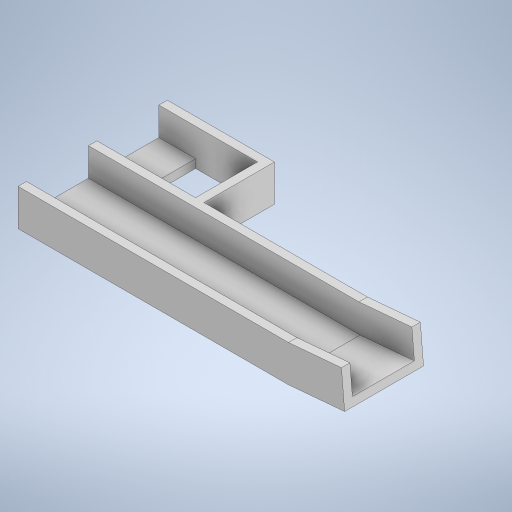
# Autodesk Inventor part: Trilho 5 min
Saved by Autodesk Inventor 2024 (Build 280153020, 153B)
## iProperties
Created: 2023-05-22
Part Number: Trilho 5 min
Material: Genérico
Document SubType Name: Modeling
Designer: jpjoa
Density: 1 g/cm^3
Appearance: Padrão
Author: jpjoa
Autodesk Inventor part; units mm, degrees
ref_plane "YZ Plane" through (0, 0, 0) normal (1, 0, 0) x (0, 1, 0)
ref_plane "XZ Plane" through (0, 0, 0) normal (0, 1, 0) x (-1, 0, 0)
sketch "Esboço1" plane through (0, 0, 0) normal (0, 1, 0) x (-1, 0, 0)
  line L0 (-93, -3) -> (0, -3)
  line L1 (0, -25) -> (-58, -25)
  line L2 (-93, 0) -> (-93, -28)
  line L3 (-93, -28) -> (-83, -28)
  line L4 (-55, -28) -> (0, -28)
  line L5 (0, -28) -> (0, 0)
  line L6 (0, 0) -> (-93, 0)
  line L7 (-55, -28) -> (-55, -53)
  line L8 (-55, -53) -> (-93, -53)
  line L9 (-93, -53) -> (-93, -50)
  line L10 (-93, -50) -> (-58, -50)
  line L11 (-58, -50) -> (-58, -25)
  arc A0 (-83, -50) -> (-58, -25) centre (-83, -25) ccw
  arc A1 (-83, -28) -> (-80, -25) centre (-83, -25) ccw
  line L12 (-93, -25) -> (-80, -25)
  line L13 (0, 0) -> (3, 0)
  line L14 (3, 0) -> (3, -28)
  line L15 (3, -28) -> (0, -28)
  line L16 (-83, -28) -> (-83, -25)
  line L17 (-93, -50) -> (-93, -28)
  line L18 (0, -3) -> (3, -3)
  line L19 (0, -25) -> (3, -25)
  line L20 (-93, -3) -> (-186, -3)
  line L21 (-186, -25) -> (-128, -25)
  line L22 (-131, -28) -> (-186, -28)
  line L23 (-186, -28) -> (-186, 0)
  line L24 (-186, 0) -> (-93, 0)
  line L25 (-131, -28) -> (-131, -53)
  line L26 (-131, -53) -> (-93, -53)
  line L27 (-93, -50) -> (-128, -50)
  line L28 (-128, -50) -> (-128, -25)
  line L29 (-186, 0) -> (-189, 0)
  line L30 (-189, 0) -> (-189, -28)
  line L31 (-189, -28) -> (-186, -28)
  line L32 (-186, -3) -> (-189, -3)
  line L33 (-186, -25) -> (-189, -25)
  line L34 (-93, -28) -> (-128, -28)
  line L35 (-93, -25) -> (-128, -25)
  line L36 (-106, -50) -> (-106, -28)
  point P0 (-93, -14)
  point P1 (-93, -51.5)
  point P2 (-83, -28)
  dimension "d7" = 22
  dimension "d9" = 3
  dimension "d10" = 3
  dimension "d13" = 3
  dimension "d14" = 3
  dimension "d16" = 22
  dimension "d20" = 22
  dimension "d21" = 80
  dimension "d29" = 3
  dimension "d31" = 10
  dimension "d39" = 22
  constraints: 74 end point, 14 point on line, 13 symmetric about line, 11 perpendicular, 6 horizontal, 4 point on circle, 3 horizontal alignment, 2 centre point, 2 coincident, 2 midpoint, 2 vertical, 2 vertical alignment, 1 collinear
  measures "d7" distance between parallel lines of L0 L1
  measures "d9" distance between parallel lines of L1 L4
  measures "d10" distance between parallel lines of L6 L0
  measures "d13" distance between parallel lines of L11 L7
  measures "d14" distance between parallel lines of L10 L8
  measures "d16" distance between parallel lines of L10 L4
  measures "d20" radial gap between concentric circles of A0 A1
  measures "d21" distance from line of L5 L12.end
  measures "d29" distance between parallel lines of L14 L5
  measures "d31" distance of L9.end A0.start
  measures "d39" distance between parallel lines of L28 L36
extrude "Extrusão1" add sketch "Esboço1" against normal blind 3 contours L20 L23 L24 L2 | L2 L35 L21 L23 L20 | L2 L34 L28 L35 | L32 L30 L29 L23 | L23 L33 L30 L32 | L17 L27 L36 L34 | L28 L27 L9 L26 L25 L22 L23 L21 | L23 L31 L30 L33
extrude "Extrusão2" add sketch "Esboço1" along normal blind 10 contours L20 L23 L24 L2 | L2 L34 L28 L35 | L32 L30 L29 L23 | L28 L27 L9 L26 L25 L22 L23 L21 | L23 L31 L30 L33
sketch "Esboço2" plane through (93, -3, 0) normal (0, 0, 1) x (1, 0, 0)
  line L0 (0, 13) -> (96, 13) projected
  line L1 (96, 0) -> (0, 0) projected
  line L2 (96, 0) -> (115.9239, 1.7431)
  line L3 (96, 0) -> (116, 0) construction
  line L4 (115.9239, 1.7431) -> (114.7952, 14.6444)
  line L5 (114.7952, 14.6444) -> (96, 13)
  line L6 (96, 0) -> (96, 13) projected
  line L7 (96, 0) -> (96, 13)
  dimension "d32" = 20
  dimension "d33" = 5
  constraints: 10 end point, 2 perpendicular, 1 equal length, 1 horizontal, 1 vertical
  measures "d32" distance of L1.start L2.end
  measures "d33" angle of L3 L2
extrude "Extrusão4" add sketch "Esboço2" against normal up to surface (28 mm away)
ref_plane "Plano de trabalho1" through (131, -3, -14) normal (0, 0, -1) x (-1, 0, 0)
sketch "Esboço3" plane through (131, -3, -14) normal (0, 0, -1) x (-1, 0, 0)
  line L0 (-76.7952, 14.6444) -> (-58, 13) projected
  line L1 (38, 13) -> (-58, 13) projected
  line L2 (-77.6667, 4.6824) -> (-58.4366, 3)
  line L3 (-58.4366, 3) -> (38, 3)
  line L4 (-77.9239, 1.7431) -> (-76.7952, 14.6444) projected
  line L5 (-76.7952, 14.6444) -> (-77.6667, 4.6824)
  line L6 (-58, 3) -> (-58, 13) projected
  line L7 (-76.7952, 14.6444) -> (-58, 13)
  line L8 (-58, 13) -> (-58, 3)
  dimension "d40" = 10
  constraints: 10 end point, 2 collinear, 1 other
  measures "d40" distance between parallel lines of L0 L2
extrude "Extrusão5" cut sketch "Esboço3" along normal mid plane 22
equation "\"d9\" = mdf"
equation "\"d10\" = mdf"
equation "\"d13\" = mdf"
equation "\"d14\" = mdf"
equation "\"mdf\" = 3"
equation "\"margem\" = 1"
